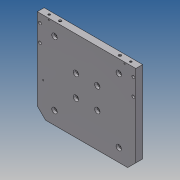
# Autodesk Inventor part: J008085
Saved by Autodesk Inventor 2018.3 (Build 223284000, 284)
## iProperties
Created: 2019-09-03
Material: ALUMINUM, 6061-T651
Vendor: HHMI: JRC - ID&F
Document SubType Name: Modeling
Designer: arnoldj
Density: 2.7 g/cm^3
Appearance: Metal-AL-6061 (Machined)
Part Number: J008085
Project: COMMON
Description: BBP Z STAGE MOUNTING PLATE
RuleStatus: InUse
AfterDocSave0: file://Part Number Cleaner
LAB/DEPT: COMMON
REQUESTING SCIENTIST: COMMON
SURFACE ROUGHNESS: 63 Ra
DESIGN DEPARTMENT: HHMI: JRC - ID&F
SPECIAL FINISH: ANODIZE PER MIL-A-8625F, TYPE II, CLASS 2 (BLACK)
ALTERED ITEM PART NUMBER: N/A
ALTERED ITEM VENDOR: N/A
ALTERED ITEM DESCRIPTION: N/A
Author: arnoldj
Revision Number: -
Autodesk Inventor part; units mm, degrees
ref_plane "YZ Plane" through (0, 0, 0) normal (1, 0, 0) x (0, 1, 0)
ref_plane "XZ Plane" through (0, 0, 0) normal (0, 1, 0) x (-1, 0, 0)
ref_plane "XY Plane" through (0, 0, 0) normal (0, 0, 1) x (1, 0, 0)
sketch "Sketch1" plane through (0, 0, 0) normal (0, 0, 1) x (1, 0, 0)
  line L0 (0, 147) -> (0, -147) projected
  line L1 (-161, 0) -> (161, 0) projected
  line L2 (115, -105) -> (-115, -105)
  line L3 (-115, -105) -> (-115, 105)
  line L4 (-115, 105) -> (115, 105)
  line L5 (115, 105) -> (115, -105)
  line L6 (115, -105) -> (-115, 105) construction
  line L7 (-115, -105) -> (115, 105) construction
  line L8 (75, -75) -> (-75, -75) construction
  line L9 (-75, -75) -> (-75, 75) construction
  line L10 (-75, 75) -> (75, 75) construction
  line L11 (75, 75) -> (75, -75) construction
  line L12 (75, -75) -> (-75, 75) construction
  line L13 (-75, -75) -> (75, 75) construction
  line L14 (25, -25) -> (-25, -25) construction
  line L15 (-25, -25) -> (-25, 25) construction
  line L16 (-25, 25) -> (25, 25) construction
  line L17 (25, 25) -> (25, -25) construction
  line L18 (25, -25) -> (-25, 25) construction
  line L19 (-25, -25) -> (25, 25) construction
  point P0 (0, 0)
  dimension "d0" = 230
  dimension "d1" = 210
  dimension "d2" = 150
  dimension "d3" = 150
  dimension "d4" = 50
  dimension "d5" = 50
  constraints: 36 end point, 8 coincident, 6 midpoint, 6 parallel, 3 horizontal, 3 perpendicular
  measures "d0" distance of L3.end L4.end
  measures "d1" distance of L2.end L3.end
  measures "d2" distance of L9.end L10.end
  measures "d3" distance of L8.end L9.end
  measures "d4" distance of L15.end L16.end
  measures "d5" distance of L14.end L15.end
extrude "Extrusion1" add sketch "Sketch1" against normal blind 15.875
hole "Hole1" at (-75, 75, 0) at (75, 75, 0) at (75, -75, 0) at (-75, -75, 0) at (-25, 25, 0) at (25, 25, 0) at (25, -25, 0) at (-25, -25, 0) direction (0, 0, -1) diameter 7.0104 end through all counterbore diameter 12.7 counterbore depth 5.9944 clearance for "Socket Head Cap Screw" size "M6" standard "Ansi Metric M Profile"
sketch "Sketch2" plane through (0, 0, -15.875) normal (0, 0, -1) x (-1, 0, 0)
  line L0 (0, -147) -> (0, 147) projected
  line L1 (-161, 0) -> (161, 0) projected
  line L2 (100, -100) -> (-100, -100) construction
  line L3 (-100, -100) -> (-100, 100) construction
  line L4 (-100, 100) -> (100, 100) construction
  line L5 (100, 100) -> (100, -100) construction
  line L6 (100, -100) -> (-100, 100) construction
  line L7 (-100, -100) -> (100, 100) construction
  circle A0 centre (101.5, -27) radius 1.5 construction
  circle A1 centre (88.57, 101.5) radius 1.5 construction
  circle A2 centre (-88.57, 101.5) radius 1.5 construction
  point P0 (0, 0)
  dimension "d15" = 200
  dimension "d16" = 200
  dimension "d17" = 3
  dimension "d18" = 127
  dimension "d19" = 11.43
  dimension "d20" = 11.43
  constraints: 12 end point, 3 centre point, 3 tangent, 2 equal radius, 2 midpoint, 2 parallel, 1 horizontal, 1 perpendicular
  measures "d15" distance of L3.end L4.end
  measures "d16" distance of L2.end L3.end
  measures "d17" diameter of A0
  measures "d18" distance from line of L4 A0.centre
  measures "d19" distance from line of A1.centre L5
  measures "d20" distance from line of L3 A2.centre
hole "Hole2" at (-101.5, -27, -15.875) at (-88.57, 101.5, -15.875) at (88.57, 101.5, -15.875) direction (0, 0, 1) diameter 2.9972 end through all counterbore diameter 3.0226 counterbore depth 1.905
chamfer "Chamfer1" distance 19.05 angle 45 2 edges at (-115, -105, -7.9375) (115, -105, -7.9375)
sketch "Sketch3" plane through (-115, 105, 0) normal (0, 1, 0) x (1, 0, 0)
  line L0 (115, 19.05) -> (115, -3.175) projected
  line L1 (276, 0) -> (-46, 0) projected
  line L2 (19.75, 7.9375) -> (210.25, 7.9375) construction
  line L3 (0, 15.875) -> (230, 15.875) projected
  point P0 (115, 0)
  point P1 (45.15, 7.9375)
  point P2 (184.85, 7.9375)
  dimension "d31" = 95.25
  dimension "d32" = 95.25
  dimension "d33" = 69.85
  dimension "d34" = 69.85
  dimension "d49" = 7.9375
  dimension "d50" = 15.875
  constraints: 2 coincident, 2 end point, 2 point on line, 1 horizontal
  measures "d31" distance from line of L0 point (210.25, 7.938)
  measures "d32" distance from line of L0 point (19.75, 7.938)
  measures "d33" distance from line of L0 point (184.85, 7.938)
  measures "d34" distance from line of L0 point (45.15, 7.938)
  measures "d49" distance between parallel lines of L2 L1
  measures "d50" distance between parallel lines of L1 L3
hole "Hole3" at (95.25, 105, -7.9375) at (-95.25, 105, -7.9375) direction (0, -1, 0) diameter 4.9276 depth 12.7 tip angle 118
hole "Hole4" at (69.85, 105, -7.9375) at (-69.85, 105, -7.9375) direction (0, -1, 0) diameter 6.35 depth 12.7 tip angle 118 counterbore diameter 6.3754 counterbore depth 3.175
sketch "Sketch4" plane through (0, 0, 0) normal (0, 0, 1) x (1, 0, 0)
  line L0 (0, 147) -> (0, -147) projected
  line L1 (-161, 0) -> (161, 0) projected
  line L2 (-115, -85.95) -> (-115, 105) projected
  line L3 (115, 105) -> (115, -85.95) projected
  line L4 (109, 45) -> (-109, 45) construction
  line L5 (-109, 45) -> (-109, 85) construction
  line L6 (-109, 85) -> (109, 85) construction
  line L7 (109, 85) -> (109, 45) construction
  line L8 (109, 45) -> (-109, 85) construction
  line L9 (-109, 45) -> (109, 85) construction
  line L10 (-115, 105) -> (115, 105) construction
  point P0 (0, 0)
  point P1 (0, 65)
  dimension "d51" = 6
  dimension "d52" = 20
  dimension "d53" = 40
  constraints: 12 end point, 4 coincident, 2 midpoint, 2 parallel, 1 horizontal, 1 perpendicular, 1 point on line
  measures "d51" distance between parallel lines of L2 L5
  measures "d52" distance between parallel lines of L6 L10
  measures "d53" distance of L4.end L5.end
hole "Hole5" at (-109, 85, 0) at (-109, 45, 0) at (109, 45, 0) at (109, 85, 0) direction (0, 0, -1) diameter 6.604 end through all clearance for "Socket Head Cap Screw" size "M6" standard "Ansi Metric M Profile"
equation "\"d32\" = d31"
equation "\"d34\" = d33"
equation "\"d49\" = 0.5 * d50"
body "Solid1"
